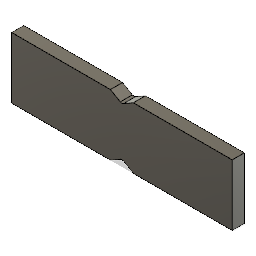
Table_17p1_Problem_2 (Autodesk Fusion 360 design; units mm, degrees)
Autodesk Fusion 360 part; units mm, degrees
sketch "Sketch1" plane through (0, 0, 0) normal (0, 0, 1) x (1, 0, 0)
  line L0 (-90, 0) -> (-90, 25)
  line L1 (-90, 25) -> (-9.3301, 25)
  line L2 (-9.3301, 25) -> (-1.25, 20.3349)
  arc A0 (-1.25, 20.3349) -> (1.25, 20.3349) centre (0, 22.5) ccw
  line L3 (1.25, 20.3349) -> (9.3301, 25)
  line L4 (9.3301, 25) -> (90, 25)
  line L5 (90, 25) -> (90, 0)
  line L6 (-90, 0) -> (90, 0) construction
  line L7 (0, 0) -> (0, 22.5) construction
  line L8 (-90, 0) -> (-90, -25)
  line L9 (-90, -25) -> (-9.3301, -25)
  line L10 (-9.3301, -25) -> (-1.25, -20.3349)
  line L11 (1.25, -20.3349) -> (9.3301, -25)
  line L12 (9.3301, -25) -> (90, -25)
  line L13 (90, -25) -> (90, 0)
  arc A1 (1.25, -20.3349) -> (-1.25, -20.3349) centre (0, -22.5) ccw
  line L14 (-90, 20) -> (90, 20) construction
  dimension "Total_Width" = 180
  dimension "Notch_Radius" = 2.5
  dimension "Notch_Theta" = 120
  dimension "Total_Height" = 50
  dimension "Notch_Height" = 5
  constraint vertical L0
  constraint perpendicular L0 L1
  constraint tangent L2 A0
  constraint horizontal L4
  constraint perpendicular L4 L5
  constraint perpendicular L5 L6
  constraint coincident L7.start origin
  constraint coincident A0.centre L7.end
  constraint vertical L7
  constraint tangent A0 L3
  constraint equal L2 L3
  constraint equal L1 L4
  constraint equal L0 L5
  constraint symmetric L0.start L6 L8.start
  constraint symmetric L0.end L6 L8.end
  constraint symmetric L1.end L6 L9.end
  constraint symmetric L2.end L6 L10.end
  constraint symmetric A0.end L6 L11.start
  constraint symmetric A0 L6 A1
  constraint symmetric L3.end L6 L11.end
  constraint symmetric L4.end L6 L12.end
  constraint symmetric L5.end L6 L13.end
  constraint coincident L7.start L6
  constraint coincident L0 L14.start
  constraint coincident L5 L14.end
  constraint horizontal L14
  constraint tangent A0 L14
  measures "Total_Width" distance of L0.start L5.end
  measures "Notch_Radius" radius of A0
  measures "Notch_Theta" angle of L2 L3
  measures "Total_Height" distance of L1 L9
  measures "Notch_Height" distance of L1 L14
extrude "Extrude1" add sketch "Sketch1" along normal mid plane 10
equation "Thickness = 1 cm"
